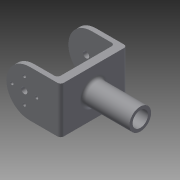
# Autodesk Inventor part: Pen
Saved by Autodesk Inventor 2015 (Build 190159000, 159)
## iProperties
Created: 2016-11-30
Part Number: Pen
Material: Generic
Document SubType Name: Modeling
Designer: Rudge-Top
Density: 1 g/cm^3
Appearance: Default
Author: Rudge-Top
Autodesk Inventor part; units mm, degrees
ref_plane "YZ Plane" through (0, 0, 0) normal (1, 0, 0) x (0, 1, 0)
ref_plane "XZ Plane" through (0, 0, 0) normal (0, 1, 0) x (-1, 0, 0)
ref_plane "XY Plane" through (0, 0, 0) normal (0, 0, 1) x (1, 0, 0)
sketch "Sketch1" plane through (0, 0, 0) normal (0, 1, 0) x (-1, 0, 0)
  line L0 (0, 0) -> (30, 0)
  line L1 (0, 0) -> (0, -37)
  line L2 (0, -37) -> (30, -37)
  line L3 (30, 0) -> (30, 3)
  line L4 (30, 3) -> (-5, 3)
  line L5 (-5, 3) -> (-5, -40)
  line L6 (-5, -40) -> (30, -40)
  line L7 (30, -40) -> (30, -37)
  dimension "d0" = 30
  dimension "d1" = 37
  dimension "d2" = 30
  dimension "d3" = 90
  dimension "d4" = 3
  dimension "d5" = 35
  dimension "d6" = 43
  constraints: 16 end point, 4 perpendicular, 2 horizontal, 2 vertical
  measures "d0" distance of L0.start L0.end
  measures "d1" distance of L0.start L1.end
  measures "d2" distance of L1.end L2.end
  measures "d3" angle of L2 L1
  measures "d4" distance of L0.end L3.end
  measures "d5" distance of L3.end L4.end
  measures "d6" distance of L4.end L5.end
extrude "Extrusion1" add sketch "Sketch1" along normal blind 30
fillet "Fillet1" radius 2 4 edges at (5, 15, 3) (5, 15, -40) (0, 15, -37) (0, 15, 0)
sketch "Sketch2" plane through (5, 0, 1) normal (1, 0, 0) x (0, 0, -1)
  line L0 (39, 30) -> (39, 0) projected
  line L1 (0, 30) -> (39, 30) projected
  line L2 (0, 0) -> (0, 30) projected
  line L3 (0, 0) -> (39, 0) projected
  circle A0 centre (19.5, 15) radius 5
  circle A1 centre (19.5, 15) radius 7
  point P0 (1, 0)
  dimension "d10" = 10
  dimension "d11" = 14
  constraints: 2 centre point, 1 coincident
  measures "d10" diameter of A0
  measures "d11" diameter of A1
extrude "Extrusion2" add sketch "Sketch2" along normal blind 30 contours A1
fillet "Fillet2" radius 2 1 edges at (5, 15, -11.5)
fillet "Fillet3" radius 15 4 edges at (-30, 30, 1.5) (-30, 0, 1.5) (-30, 30, -38.5) (-30, 0, -38.5)
sketch "Sketch3" plane through (3, 0, 3) normal (0, 0, 1) x (1, 0, 0)
  arc A0 (-18, 30) -> (-18, 0) centre (-18, 15) ccw projected
  line L0 (-18, 0) -> (0, 0) projected
  line L1 (0, 30) -> (0, 0) projected
  line L2 (-18, 30) -> (0, 30) projected
  circle A1 centre (-21.5, 15) radius 11
  point P0 (-3, 0)
  point P1 (-29.5, 15)
  point P2 (-21.5, 23)
  point P3 (-13.5, 15)
  point P4 (-21.5, 7)
  dimension "d16" = 22
  dimension "d18" = 8
  dimension "d19" = 8
  dimension "d20" = 8
  dimension "d21" = 8
  constraints: 1 centre point, 1 coincident
  measures "d16" diameter of A1
  measures "d18" distance of A1.centre point (-13.5, 15)
  measures "d19" distance of point (-29.5, 15) point (-21.5, 15)
  measures "d20" distance of point (-21.5, 15) point (-21.5, 7)
  measures "d21" distance of point (-21.5, 15) point (-21.5, 23)
hole "Hole1" at (-18.5, 15, 3) at (-26.5, 15, 3) at (-18.5, 23, 3) at (-10.5, 15, 3) at (-18.5, 7, 3) direction (0, 0, -1) diameter 2 depth 8 tip angle 118
sketch "Sketch4" plane through (3, 0, -40) normal (0, 0, -1) x (-1, 0, 0)
  circle A0 centre (13.5, 15) radius 1 projected
  circle A1 centre (29.5, 15) radius 1 projected
  circle A2 centre (21.5, 15) radius 1 projected
  circle A3 centre (21.5, 23) radius 1 projected
  circle A4 centre (21.5, 7) radius 1 projected
  arc A5 (18, 0) -> (18, 30) centre (18, 15) ccw projected
  line L0 (5, 30) -> (18, 30) projected
  line L1 (5, 0) -> (5, 30) projected
  line L2 (5, 0) -> (18, 0) projected
  point P0 (3, 0)
  constraints: 1 coincident
hole "Hole2" at (-18.5, 15, -40) direction (0, 0, 1) diameter 4 end through all
body "Solid1"
